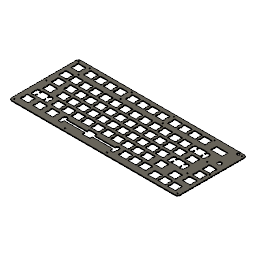
Plate (Autodesk Fusion 360 design; units mm, degrees)
part number: 2026-06-20-08-16-56-119
Autodesk Fusion 360 part; units mm, degrees
(part 1 of 6)
derive "DerivedContext1"
sketch "Sketch3" plane through (0, 0, 0) normal (0, 0, 1) x (1, 0, 0)
  line L0 (324.2389, -5.001) -> (324.612, -5.015)
  line L1 (324.612, -5.015) -> (324.9851, -5.059)
  line L2 (324.9851, -5.059) -> (325.3502, -5.132)
  line L3 (325.3502, -5.132) -> (325.71, -5.234)
  line L4 (325.71, -5.234) -> (326.0619, -5.363)
  line L5 (326.0619, -5.363) -> (326.4006, -5.52)
  line L6 (326.4006, -5.52) -> (326.726, -5.702)
  line L7 (326.726, -5.702) -> (327.0382, -5.91)
  line L8 (327.0382, -5.91) -> (327.3319, -6.142)
  line L9 (327.3319, -6.142) -> (327.6071, -6.395)
  line L10 (327.6071, -6.395) -> (327.8611, -6.67)
  line L11 (327.8611, -6.67) -> (328.0913, -6.964)
  line L12 (328.0913, -6.964) -> (328.3003, -7.275)
  line L13 (328.3003, -7.275) -> (328.4829, -7.601)
  line L14 (328.4829, -7.601) -> (328.639, -7.94)
  line L15 (328.639, -7.94) -> (328.7686, -8.291)
  line L16 (328.7686, -8.291) -> (328.8691, -8.651)
  line L17 (328.8691, -8.651) -> (328.9432, -9.018)
  line L18 (328.9432, -9.018) -> (328.9882, -9.389)
  line L19 (328.9882, -9.389) -> (329.0014, -9.763)
  line L20 (329.0014, -9.763) -> (329.0014, -133.7389)
  line L21 (329.0014, -133.7389) -> (328.9882, -134.1131)
  line L22 (328.9882, -134.1131) -> (328.9432, -134.484)
  line L23 (328.9432, -134.484) -> (328.8691, -134.851)
  line L24 (328.8691, -134.851) -> (328.7686, -135.2111)
  line L25 (328.7686, -135.2111) -> (328.639, -135.5619)
  line L26 (328.639, -135.5619) -> (328.4829, -135.9011)
  line L27 (328.4829, -135.9011) -> (328.3003, -136.2271)
  line L28 (328.3003, -136.2271) -> (328.0913, -136.538)
  line L29 (328.0913, -136.538) -> (327.8611, -136.8319)
  line L30 (327.8611, -136.8319) -> (327.6071, -137.1071)
  line L31 (327.6071, -137.1071) -> (327.3319, -137.36)
  line L32 (327.3319, -137.36) -> (327.0382, -137.5921)
  line L33 (327.0382, -137.5921) -> (326.726, -137.8)
  line L34 (326.726, -137.8) -> (326.4006, -137.9821)
  line L35 (326.4006, -137.9821) -> (326.0619, -138.139)
  line L36 (326.0619, -138.139) -> (325.71, -138.2681)
  line L37 (325.71, -138.2681) -> (325.3502, -138.3699)
  line L38 (325.3502, -138.3699) -> (324.9851, -138.443)
  line L39 (324.9851, -138.443) -> (324.612, -138.4869)
  line L40 (324.612, -138.4869) -> (324.2389, -138.502)
  line L41 (324.2389, -138.502) -> (9.763, -138.5009)
  line L42 (9.763, -138.5009) -> (9.389, -138.4869)
  line L43 (9.389, -138.4869) -> (9.018, -138.443)
  line L44 (9.018, -138.443) -> (8.651, -138.3699)
  line L45 (8.651, -138.3699) -> (8.291, -138.2681)
  line L46 (8.291, -138.2681) -> (7.94, -138.139)
  line L47 (7.94, -138.139) -> (7.601, -137.9821)
  line L48 (7.601, -137.9821) -> (7.275, -137.8)
  line L49 (7.275, -137.8) -> (6.964, -137.5921)
  line L50 (6.964, -137.5921) -> (6.67, -137.36)
  line L51 (6.67, -137.36) -> (6.395, -137.1071)
  line L52 (6.395, -137.1071) -> (6.142, -136.8319)
  line L53 (6.142, -136.8319) -> (5.91, -136.538)
  line L54 (5.91, -136.538) -> (5.702, -136.2271)
  line L55 (5.702, -136.2271) -> (5.52, -135.9011)
  line L56 (5.52, -135.9011) -> (5.363, -135.5619)
  line L57 (5.363, -135.5619) -> (5.234, -135.2111)
  line L58 (5.234, -135.2111) -> (5.132, -134.851)
  line L59 (5.132, -134.851) -> (5.059, -134.484)
  line L60 (5.059, -134.484) -> (5.015, -134.1131)
  line L61 (5.015, -134.1131) -> (5, -133.7389)
  line L62 (5, -133.7389) -> (5.001, -9.763)
  line L63 (5.001, -9.763) -> (5.015, -9.389)
  line L64 (5.015, -9.389) -> (5.059, -9.018)
  line L65 (5.059, -9.018) -> (5.132, -8.651)
  line L66 (5.132, -8.651) -> (5.234, -8.291)
  line L67 (5.234, -8.291) -> (5.363, -7.94)
  line L68 (5.363, -7.94) -> (5.52, -7.601)
  line L69 (5.52, -7.601) -> (5.702, -7.275)
  line L70 (5.702, -7.275) -> (5.91, -6.964)
  line L71 (5.91, -6.964) -> (6.142, -6.67)
  line L72 (6.142, -6.67) -> (6.395, -6.395)
  line L73 (6.395, -6.395) -> (6.67, -6.142)
  line L74 (6.67, -6.142) -> (6.964, -5.91)
  line L75 (6.964, -5.91) -> (7.275, -5.702)
  line L76 (7.275, -5.702) -> (7.601, -5.52)
  line L77 (7.601, -5.52) -> (7.94, -5.363)
  line L78 (7.94, -5.363) -> (8.291, -5.234)
  line L79 (8.291, -5.234) -> (8.651, -5.132)
  line L80 (8.651, -5.132) -> (9.018, -5.059)
  line L81 (9.018, -5.059) -> (9.389, -5.015)
  line L82 (9.389, -5.015) -> (9.763, -5)
  line L83 (9.763, -5) -> (324.2389, -5.001)
  line L84 (264.8506, -117.2131) -> (264.8506, -118.2129)
  line L85 (264.8506, -118.2129) -> (264.0499, -118.2129)
  line L86 (264.0499, -118.2129) -> (264.0499, -121.163)
  line L87 (264.0499, -121.163) -> (264.8506, -121.163)
  line L88 (264.8506, -121.163) -> (264.8506, -127.113)
  line L89 (264.8506, -127.113) -> (264.0499, -127.113)
  line L90 (264.0499, -127.113) -> (264.0499, -130.0631)
  line L91 (264.0499, -130.0631) -> (264.8506, -130.0631)
  line L92 (264.8506, -130.0631) -> (264.8506, -131.0629)
  line L93 (264.8506, -131.0629) -> (278.7015, -131.0629)
  line L94 (278.7015, -131.0629) -> (278.7015, -130.0631)
  line L95 (278.7015, -130.0631) -> (279.5005, -130.0631)
  line L96 (279.5005, -130.0631) -> (279.5005, -127.113)
  line L97 (279.5005, -127.113) -> (278.7015, -127.113)
  line L98 (278.7015, -127.113) -> (278.7015, -121.163)
  line L99 (278.7015, -121.163) -> (279.5005, -121.163)
  line L100 (279.5005, -121.163) -> (279.5005, -118.2129)
  line L101 (279.5005, -118.2129) -> (278.7015, -118.2129)
  line L102 (278.7015, -118.2129) -> (278.7015, -117.2131)
  line L103 (278.7015, -117.2131) -> (264.8506, -117.2131)
  line L104 (283.9006, -117.2131) -> (283.9006, -118.2129)
  line L105 (283.9006, -118.2129) -> (283.0989, -118.2129)
  line L106 (283.0989, -118.2129) -> (283.0989, -121.163)
  line L107 (283.0989, -121.163) -> (283.9006, -121.163)
  line L108 (283.9006, -121.163) -> (283.9006, -127.113)
  line L109 (283.9006, -127.113) -> (283.0989, -127.113)
  line L110 (283.0989, -127.113) -> (283.0989, -130.0631)
  line L111 (283.0989, -130.0631) -> (283.9006, -130.0631)
  line L112 (283.9006, -130.0631) -> (283.9006, -131.0629)
  line L113 (283.9006, -131.0629) -> (297.7515, -131.0629)
  line L114 (297.7515, -131.0629) -> (297.7515, -130.0631)
  line L115 (297.7515, -130.0631) -> (298.5505, -130.0631)
  line L116 (298.5505, -130.0631) -> (298.5505, -127.113)
  line L117 (298.5505, -127.113) -> (297.7515, -127.113)
  line L118 (297.7515, -127.113) -> (297.7515, -121.163)
  line L119 (297.7515, -121.163) -> (298.5505, -121.163)
  line L120 (298.5505, -121.163) -> (298.5505, -118.2129)
  line L121 (298.5505, -118.2129) -> (297.7515, -118.2129)
  line L122 (297.7515, -118.2129) -> (297.7515, -117.2131)
  line L123 (297.7515, -117.2131) -> (283.9006, -117.2131)
  line L124 (302.9506, -117.2131) -> (302.9506, -118.2129)
  line L125 (302.9506, -118.2129) -> (302.1515, -118.2129)
  line L126 (302.1515, -118.2129) -> (302.1515, -121.163)
  line L127 (302.1515, -121.163) -> (302.9506, -121.163)
  line L128 (302.9506, -121.163) -> (302.9506, -127.113)
  line L129 (302.9506, -127.113) -> (302.1515, -127.113)
  line L130 (302.1515, -127.113) -> (302.1515, -130.0631)
  line L131 (302.1515, -130.0631) -> (302.9506, -130.0631)
  line L132 (302.9506, -130.0631) -> (302.9506, -131.0629)
  line L133 (302.9506, -131.0629) -> (316.8015, -131.0629)
  line L134 (316.8015, -131.0629) -> (316.8015, -130.0631)
  line L135 (316.8015, -130.0631) -> (317.6005, -130.0631)
  line L136 (317.6005, -130.0631) -> (317.6005, -127.113)
  line L137 (317.6005, -127.113) -> (316.8015, -127.113)
  line L138 (316.8015, -127.113) -> (316.8015, -121.163)
  line L139 (316.8015, -121.163) -> (317.6005, -121.163)
  line L140 (317.6005, -121.163) -> (317.6005, -118.2129)
  line L141 (317.6005, -118.2129) -> (316.8015, -118.2129)
  line L142 (316.8015, -118.2129) -> (316.8015, -117.2131)
  line L143 (316.8015, -117.2131) -> (302.9506, -117.2131)
  line L144 (133.8821, -112.4511) -> (133.8821, -113.4509)
  line L145 (133.8821, -113.4509) -> (133.082, -113.4509)
  line L146 (133.082, -113.4509) -> (133.082, -116.4011)
  line L147 (133.082, -116.4011) -> (133.8821, -116.4011)
  line L148 (133.8821, -116.4011) -> (133.8821, -117.1509)
  line L149 (133.8821, -117.1509) -> (94.107, -117.1509)
  line L150 (94.107, -117.1509) -> (94.107, -113.9211)
  line L151 (94.107, -113.9211) -> (92.3819, -113.9211)
  line L152 (92.3819, -113.9211) -> (92.3819, -113.0009)
  line L153 (92.3819, -113.0009) -> (89.2321, -113.0009)
  line L154 (89.2321, -113.0009) -> (89.2321, -113.9211)
  line L155 (89.2321, -113.9211) -> (87.507, -113.9211)
  line L156 (87.507, -113.9211) -> (87.507, -117.1509)
  line L157 (87.507, -117.1509) -> (86.682, -117.1509)
  line L158 (86.682, -117.1509) -> (86.682, -119.8009)
  line L159 (86.682, -119.8009) -> (87.507, -119.8009)
  line L160 (87.507, -119.8009) -> (87.507, -126.0711)
  line L161 (87.507, -126.0711) -> (89.2321, -126.0711)
  line L162 (89.2321, -126.0711) -> (89.2321, -127.0511)
  line L163 (89.2321, -127.0511) -> (92.3819, -127.0511)
  line L164 (92.3819, -127.0511) -> (92.3819, -126.0711)
  line L165 (92.3819, -126.0711) -> (94.107, -126.0711)
  line L166 (94.107, -126.0711) -> (94.107, -121.6009)
  line L167 (94.107, -121.6009) -> (133.8821, -121.6009)
  line L168 (133.8821, -121.6009) -> (133.8821, -122.351)
  line L169 (133.8821, -122.351) -> (133.082, -122.351)
  line L170 (133.082, -122.351) -> (133.082, -125.3011)
  line L171 (133.082, -125.3011) -> (133.8821, -125.3011)
  line L172 (133.8821, -125.3011) -> (133.8821, -126.301)
  line L173 (133.8821, -126.301) -> (147.732, -126.301)
  line L174 (147.732, -126.301) -> (147.732, -125.3011)
  line L175 (147.732, -125.3011) -> (148.5321, -125.3011)
  line L176 (148.5321, -125.3011) -> (148.5321, -122.351)
  line L177 (148.5321, -122.351) -> (147.732, -122.351)
  line L178 (147.732, -122.351) -> (147.732, -121.6009)
  line L179 (147.732, -121.6009) -> (187.507, -121.6009)
  line L180 (187.507, -121.6009) -> (187.507, -126.0711)
  line L181 (187.507, -126.0711) -> (189.2321, -126.0711)
  line L182 (189.2321, -126.0711) -> (189.2321, -127.0511)
  line L183 (189.2321, -127.0511) -> (192.382, -127.0511)
  line L184 (192.382, -127.0511) -> (192.382, -126.0711)
  line L185 (192.382, -126.0711) -> (194.1071, -126.0711)
  line L186 (194.1071, -126.0711) -> (194.1071, -119.8009)
  line L187 (194.1071, -119.8009) -> (194.932, -119.8009)
  line L188 (194.932, -119.8009) -> (194.932, -117.1509)
  line L189 (194.932, -117.1509) -> (194.1071, -117.1509)
  line L190 (194.1071, -117.1509) -> (194.1071, -113.9211)
  line L191 (194.1071, -113.9211) -> (192.382, -113.9211)
  line L192 (192.382, -113.9211) -> (192.382, -113.0009)
  line L193 (192.382, -113.0009) -> (189.2321, -113.0009)
  line L194 (189.2321, -113.0009) -> (189.2321, -113.9211)
  line L195 (189.2321, -113.9211) -> (187.507, -113.9211)
  line L196 (187.507, -113.9211) -> (187.507, -117.1509)
  line L197 (187.507, -117.1509) -> (147.732, -117.1509)
  line L198 (147.732, -117.1509) -> (147.732, -116.4011)
  line L199 (147.732, -116.4011) -> (148.5321, -116.4011)
  line L200 (148.5321, -116.4011) -> (148.5321, -113.4509)
  line L201 (148.5321, -113.4509) -> (147.732, -113.4509)
  line L202 (147.732, -113.4509) -> (147.732, -112.4511)
  line L203 (147.732, -112.4511) -> (133.8821, -112.4511)
  line L204 (14.819, -112.4511) -> (14.819, -113.4509)
  line L205 (14.819, -113.4509) -> (14.019, -113.4509)
  line L206 (14.019, -113.4509) -> (14.019, -116.4011)
  line L207 (14.019, -116.4011) -> (14.819, -116.4011)
  line L208 (14.819, -116.4011) -> (14.819, -122.351)
  line L209 (14.819, -122.351) -> (14.019, -122.351)
  line L210 (14.019, -122.351) -> (14.019, -125.3011)
  line L211 (14.019, -125.3011) -> (14.819, -125.3011)
  line L212 (14.819, -125.3011) -> (14.819, -126.301)
  line L213 (14.819, -126.301) -> (28.6689, -126.301)
  line L214 (28.6689, -126.301) -> (28.6689, -125.3011)
  line L215 (28.6689, -125.3011) -> (29.469, -125.3011)
  line L216 (29.469, -125.3011) -> (29.469, -122.351)
  line L217 (29.469, -122.351) -> (28.6689, -122.351)
  line L218 (28.6689, -122.351) -> (28.6689, -116.4011)
  line L219 (28.6689, -116.4011) -> (29.469, -116.4011)
  line L220 (29.469, -116.4011) -> (29.469, -113.4509)
  line L221 (29.469, -113.4509) -> (28.6689, -113.4509)
  line L222 (28.6689, -113.4509) -> (28.6689, -112.4511)
  line L223 (28.6689, -112.4511) -> (14.819, -112.4511)
  line L224 (38.6321, -112.4511) -> (38.6321, -113.4509)
  line L225 (38.6321, -113.4509) -> (37.832, -113.4509)
  line L226 (37.832, -113.4509) -> (37.832, -116.4011)
  line L227 (37.832, -116.4011) -> (38.6321, -116.4011)
  line L228 (38.6321, -116.4011) -> (38.6321, -122.351)
  line L229 (38.6321, -122.351) -> (37.832, -122.351)
  line L230 (37.832, -122.351) -> (37.832, -125.3011)
  line L231 (37.832, -125.3011) -> (38.6321, -125.3011)
  line L232 (38.6321, -125.3011) -> (38.6321, -126.301)
  line L233 (38.6321, -126.301) -> (52.482, -126.301)
  line L234 (52.482, -126.301) -> (52.482, -125.3011)
  line L235 (52.482, -125.3011) -> (53.2821, -125.3011)
  line L236 (53.2821, -125.3011) -> (53.2821, -122.351)
  line L237 (53.2821, -122.351) -> (52.482, -122.351)
  line L238 (52.482, -122.351) -> (52.482, -116.4011)
  line L239 (52.482, -116.4011) -> (53.2821, -116.4011)
  line L240 (53.2821, -116.4011) -> (53.2821, -113.4509)
  line L241 (53.2821, -113.4509) -> (52.482, -113.4509)
  line L242 (52.482, -113.4509) -> (52.482, -112.4511)
  line L243 (52.482, -112.4511) -> (38.6321, -112.4511)
  line L244 (62.444, -112.4511) -> (62.444, -113.4509)
  line L245 (62.444, -113.4509) -> (61.6439, -113.4509)
  line L246 (61.6439, -113.4509) -> (61.6439, -116.4011)
  line L247 (61.6439, -116.4011) -> (62.444, -116.4011)
  line L248 (62.444, -116.4011) -> (62.444, -122.351)
  line L249 (62.444, -122.351) -> (61.6439, -122.351)
  line L250 (61.6439, -122.351) -> (61.6439, -125.3011)
  line L251 (61.6439, -125.3011) -> (62.444, -125.3011)
  line L252 (62.444, -125.3011) -> (62.444, -126.301)
  line L253 (62.444, -126.301) -> (76.2939, -126.301)
  line L254 (76.2939, -126.301) -> (76.2939, -125.3011)
  line L255 (76.2939, -125.3011) -> (77.094, -125.3011)
  line L256 (77.094, -125.3011) -> (77.094, -122.351)
  line L257 (77.094, -122.351) -> (76.2939, -122.351)
  line L258 (76.2939, -122.351) -> (76.2939, -116.4011)
  line L259 (76.2939, -116.4011) -> (77.094, -116.4011)
  line L260 (77.094, -116.4011) -> (77.094, -113.4509)
  line L261 (77.094, -113.4509) -> (76.2939, -113.4509)
  line L262 (76.2939, -113.4509) -> (76.2939, -112.4511)
  line L263 (76.2939, -112.4511) -> (62.444, -112.4511)
  line L264 (202.9381, -112.4511) -> (202.9381, -113.4509)
  line L265 (202.9381, -113.4509) -> (202.138, -113.4509)
  line L266 (202.138, -113.4509) -> (202.138, -116.4011)
  line L267 (202.138, -116.4011) -> (202.9381, -116.4011)
  line L268 (202.9381, -116.4011) -> (202.9381, -122.351)
  line L269 (202.9381, -122.351) -> (202.138, -122.351)
  line L270 (202.138, -122.351) -> (202.138, -125.3011)
  line L271 (202.138, -125.3011) -> (202.9381, -125.3011)
  line L272 (202.9381, -125.3011) -> (202.9381, -126.301)
  line L273 (202.9381, -126.301) -> (216.7879, -126.301)
  line L274 (216.7879, -126.301) -> (216.7879, -125.3011)
  line L275 (216.7879, -125.3011) -> (217.588, -125.3011)
  line L276 (217.588, -125.3011) -> (217.588, -122.351)
  line L277 (217.588, -122.351) -> (216.7879, -122.351)
  line L278 (216.7879, -122.351) -> (216.7879, -116.4011)
  line L279 (216.7879, -116.4011) -> (217.588, -116.4011)
  line L280 (217.588, -116.4011) -> (217.588, -113.4509)
  line L281 (217.588, -113.4509) -> (216.7879, -113.4509)
  line L282 (216.7879, -113.4509) -> (216.7879, -112.4511)
  line L283 (216.7879, -112.4511) -> (202.9381, -112.4511)
  line L284 (221.9881, -112.4511) -> (221.9881, -113.4509)
  line L285 (221.9881, -113.4509) -> (221.188, -113.4509)
  line L286 (221.188, -113.4509) -> (221.188, -116.4011)
  line L287 (221.188, -116.4011) -> (221.9881, -116.4011)
  line L288 (221.9881, -116.4011) -> (221.9881, -122.351)
  line L289 (221.9881, -122.351) -> (221.188, -122.351)
  line L290 (221.188, -122.351) -> (221.188, -125.3011)
  line L291 (221.188, -125.3011) -> (221.9881, -125.3011)
  line L292 (221.9881, -125.3011) -> (221.9881, -126.301)
  line L293 (221.9881, -126.301) -> (235.8379, -126.301)
  line L294 (235.8379, -126.301) -> (235.8379, -125.3011)
  line L295 (235.8379, -125.3011) -> (236.638, -125.3011)
  line L296 (236.638, -125.3011) -> (236.638, -122.351)
  line L297 (236.638, -122.351) -> (235.8379, -122.351)
  line L298 (235.8379, -122.351) -> (235.8379, -116.4011)
  line L299 (235.8379, -116.4011) -> (236.638, -116.4011)
  line L300 (236.638, -116.4011) -> (236.638, -113.4509)
  line L301 (236.638, -113.4509) -> (235.8379, -113.4509)
  line L302 (235.8379, -113.4509) -> (235.8379, -112.4511)
  line L303 (235.8379, -112.4511) -> (221.9881, -112.4511)
  line L304 (241.0381, -112.4511) -> (241.0381, -113.4509)
  line L305 (241.0381, -113.4509) -> (240.238, -113.4509)
  line L306 (240.238, -113.4509) -> (240.238, -116.4011)
  line L307 (240.238, -116.4011) -> (241.0381, -116.4011)
  line L308 (241.0381, -116.4011) -> (241.0381, -122.351)
  line L309 (241.0381, -122.351) -> (240.238, -122.351)
  line L310 (240.238, -122.351) -> (240.238, -125.3011)
  line L311 (240.238, -125.3011) -> (241.0381, -125.3011)
  line L312 (241.0381, -125.3011) -> (241.0381, -126.301)
  line L313 (241.0381, -126.301) -> (254.8879, -126.301)
  line L314 (254.8879, -126.301) -> (254.8879, -125.3011)
  line L315 (254.8879, -125.3011) -> (255.688, -125.3011)
  line L316 (255.688, -125.3011) -> (255.688, -122.351)
  line L317 (255.688, -122.351) -> (254.8879, -122.351)
  line L318 (254.8879, -122.351) -> (254.8879, -116.4011)
  line L319 (254.8879, -116.4011) -> (255.688, -116.4011)
  line L320 (255.688, -116.4011) -> (255.688, -113.4509)
  line L321 (255.688, -113.4509) -> (254.8879, -113.4509)
  line L322 (254.8879, -113.4509) -> (254.8879, -112.4511)
  line L323 (254.8879, -112.4511) -> (241.0381, -112.4511)
  line L324 (283.9006, -98.1631) -> (283.9006, -99.1629)
  line L325 (283.9006, -99.1629) -> (283.0989, -99.1629)
  line L326 (283.0989, -99.1629) -> (283.0989, -102.113)
  line L327 (283.0989, -102.113) -> (283.9006, -102.113)
  line L328 (283.9006, -102.113) -> (283.9006, -108.063)
  line L329 (283.9006, -108.063) -> (283.0989, -108.063)
  line L330 (283.0989, -108.063) -> (283.0989, -111.0131)
  line L331 (283.0989, -111.0131) -> (283.9006, -111.0131)
  line L332 (283.9006, -111.0131) -> (283.9006, -112.0129)
  line L333 (283.9006, -112.0129) -> (297.7515, -112.0129)
  line L334 (297.7515, -112.0129) -> (297.7515, -111.0131)
  line L335 (297.7515, -111.0131) -> (298.5505, -111.0131)
  line L336 (298.5505, -111.0131) -> (298.5505, -108.063)
  line L337 (298.5505, -108.063) -> (297.7515, -108.063)
  line L338 (297.7515, -108.063) -> (297.7515, -102.113)
  line L339 (297.7515, -102.113) -> (298.5505, -102.113)
  line L340 (298.5505, -102.113) -> (298.5505, -99.1629)
  line L341 (298.5505, -99.1629) -> (297.7515, -99.1629)
  line L342 (297.7515, -99.1629) -> (297.7515, -98.1631)
  line L343 (297.7515, -98.1631) -> (283.9006, -98.1631)
  line L344 (24.344, -93.4) -> (24.344, -94.3999)
  line L345 (24.344, -94.3999) -> (23.544, -94.3999)
  line L346 (23.544, -94.3999) -> (23.544, -97.3511)
  line L347 (23.544, -97.3511) -> (24.344, -97.3511)
  line L348 (24.344, -97.3511) -> (24.344, -98.1009)
  line L349 (24.344, -98.1009) -> (22.669, -98.1009)
  line L350 (22.669, -98.1009) -> (22.669, -94.8701)
  line L351 (22.669, -94.8701) -> (20.944, -94.8701)
  line L352 (20.944, -94.8701) -> (20.944, -93.9501)
  line L353 (20.944, -93.9501) -> (17.794, -93.9501)
  line L354 (17.794, -93.9501) -> (17.794, -94.8701)
  line L355 (17.794, -94.8701) -> (16.069, -94.8701)
  line L356 (16.069, -94.8701) -> (16.069, -98.1009)
  line L357 (16.069, -98.1009) -> (15.244, -98.1009)
  line L358 (15.244, -98.1009) -> (15.244, -100.7499)
  line L359 (15.244, -100.7499) -> (16.069, -100.7499)
  line L360 (16.069, -100.7499) -> (16.069, -107.02)
  line L361 (16.069, -107.02) -> (17.794, -107.02)
  line L362 (17.794, -107.02) -> (17.794, -108)
  line L363 (17.794, -108) -> (20.944, -108)
  line L364 (20.944, -108) -> (20.944, -107.02)
  line L365 (20.944, -107.02) -> (22.669, -107.02)
  line L366 (22.669, -107.02) -> (22.669, -102.5501)
  line L367 (22.669, -102.5501) -> (24.344, -102.5501)
  line L368 (24.344, -102.5501) -> (24.344, -103.2999)
  line L369 (24.344, -103.2999) -> (23.544, -103.2999)
  line L370 (23.544, -103.2999) -> (23.544, -106.2501)
  line L371 (23.544, -106.2501) -> (24.344, -106.2501)
  line L372 (24.344, -106.2501) -> (24.344, -107.2499)
  line L373 (24.344, -107.2499) -> (38.1939, -107.2499)
  line L374 (38.1939, -107.2499) -> (38.1939, -106.2501)
  line L375 (38.1939, -106.2501) -> (38.994, -106.2501)
  line L376 (38.994, -106.2501) -> (38.994, -103.2999)
  line L377 (38.994, -103.2999) -> (38.1939, -103.2999)
  line L378 (38.1939, -103.2999) -> (38.1939, -102.5501)
  line L379 (38.1939, -102.5501) -> (39.869, -102.5501)
  line L380 (39.869, -102.5501) -> (39.869, -107.02)
  line L381 (39.869, -107.02) -> (41.5941, -107.02)
  line L382 (41.5941, -107.02) -> (41.5941, -108)
  line L383 (41.5941, -108) -> (44.744, -108)
  line L384 (44.744, -108) -> (44.744, -107.02)
  line L385 (44.744, -107.02) -> (46.469, -107.02)
  line L386 (46.469, -107.02) -> (46.469, -100.7499)
  line L387 (46.469, -100.7499) -> (47.294, -100.7499)
  line L388 (47.294, -100.7499) -> (47.294, -98.1009)
  line L389 (47.294, -98.1009) -> (46.469, -98.1009)
  line L390 (46.469, -98.1009) -> (46.469, -94.8701)
  line L391 (46.469, -94.8701) -> (44.744, -94.8701)
  line L392 (44.744, -94.8701) -> (44.744, -93.9501)
  line L393 (44.744, -93.9501) -> (41.5941, -93.9501)
  line L394 (41.5941, -93.9501) -> (41.5941, -94.8701)
  line L395 (41.5941, -94.8701) -> (39.869, -94.8701)
  line L396 (39.869, -94.8701) -> (39.869, -98.1009)
  line L397 (39.869, -98.1009) -> (38.1939, -98.1009)
  line L398 (38.1939, -98.1009) -> (38.1939, -97.3511)
  line L399 (38.1939, -97.3511) -> (38.994, -97.3511)
  line L400 (38.994, -97.3511) -> (38.994, -94.3999)
  line L401 (38.994, -94.3999) -> (38.1939, -94.3999)
  line L402 (38.1939, -94.3999) -> (38.1939, -93.4)
  line L403 (38.1939, -93.4) -> (24.344, -93.4)
  line L404 (55.3011, -93.4) -> (55.3011, -94.3999)
  line L405 (55.3011, -94.3999) -> (54.501, -94.3999)
  line L406 (54.501, -94.3999) -> (54.501, -97.3511)
  line L407 (54.501, -97.3511) -> (55.3011, -97.3511)
  line L408 (55.3011, -97.3511) -> (55.3011, -103.2999)
  line L409 (55.3011, -103.2999) -> (54.501, -103.2999)
  line L410 (54.501, -103.2999) -> (54.501, -106.2501)
  line L411 (54.501, -106.2501) -> (55.3011, -106.2501)
  line L412 (55.3011, -106.2501) -> (55.3011, -107.2499)
  line L413 (55.3011, -107.2499) -> (69.151, -107.2499)
  line L414 (69.151, -107.2499) -> (69.151, -106.2501)
  line L415 (69.151, -106.2501) -> (69.9511, -106.2501)
  line L416 (69.9511, -106.2501) -> (69.9511, -103.2999)
  line L417 (69.9511, -103.2999) -> (69.151, -103.2999)
  line L418 (69.151, -103.2999) -> (69.151, -97.3511)
  line L419 (69.151, -97.3511) -> (69.9511, -97.3511)
  line L420 (69.9511, -97.3511) -> (69.9511, -94.3999)
  line L421 (69.9511, -94.3999) -> (69.151, -94.3999)
  line L422 (69.151, -94.3999) -> (69.151, -93.4)
  line L423 (69.151, -93.4) -> (55.3011, -93.4)
  line L424 (74.3511, -93.4) -> (74.3511, -94.3999)
  line L425 (74.3511, -94.3999) -> (73.551, -94.3999)
  line L426 (73.551, -94.3999) -> (73.551, -97.3511)
  line L427 (73.551, -97.3511) -> (74.3511, -97.3511)
  line L428 (74.3511, -97.3511) -> (74.3511, -103.2999)
  line L429 (74.3511, -103.2999) -> (73.551, -103.2999)
  line L430 (73.551, -103.2999) -> (73.551, -106.2501)
  line L431 (73.551, -106.2501) -> (74.3511, -106.2501)
  line L432 (74.3511, -106.2501) -> (74.3511, -107.2499)
  line L433 (74.3511, -107.2499) -> (88.201, -107.2499)
  line L434 (88.201, -107.2499) -> (88.201, -106.2501)
  line L435 (88.201, -106.2501) -> (89.0011, -106.2501)
  line L436 (89.0011, -106.2501) -> (89.0011, -103.2999)
  line L437 (89.0011, -103.2999) -> (88.201, -103.2999)
  line L438 (88.201, -103.2999) -> (88.201, -97.3511)
  line L439 (88.201, -97.3511) -> (89.0011, -97.3511)
  line L440 (89.0011, -97.3511) -> (89.0011, -94.3999)
  line L441 (89.0011, -94.3999) -> (88.201, -94.3999)
  line L442 (88.201, -94.3999) -> (88.201, -93.4)
  line L443 (88.201, -93.4) -> (74.3511, -93.4)
  line L444 (93.4011, -93.4) -> (93.4011, -94.3999)
  line L445 (93.4011, -94.3999) -> (92.601, -94.3999)
  line L446 (92.601, -94.3999) -> (92.601, -97.3511)
  line L447 (92.601, -97.3511) -> (93.4011, -97.3511)
  line L448 (93.4011, -97.3511) -> (93.4011, -103.2999)
  line L449 (93.4011, -103.2999) -> (92.601, -103.2999)
  line L450 (92.601, -103.2999) -> (92.601, -106.2501)
  line L451 (92.601, -106.2501) -> (93.4011, -106.2501)
  line L452 (93.4011, -106.2501) -> (93.4011, -107.2499)
  line L453 (93.4011, -107.2499) -> (107.251, -107.2499)
  line L454 (107.251, -107.2499) -> (107.251, -106.2501)
  line L455 (107.251, -106.2501) -> (108.0511, -106.2501)
  line L456 (108.0511, -106.2501) -> (108.0511, -103.2999)
  line L457 (108.0511, -103.2999) -> (107.251, -103.2999)
  line L458 (107.251, -103.2999) -> (107.251, -97.3511)
  line L459 (107.251, -97.3511) -> (108.0511, -97.3511)
  line L460 (108.0511, -97.3511) -> (108.0511, -94.3999)
  line L461 (108.0511, -94.3999) -> (107.251, -94.3999)
  line L462 (107.251, -94.3999) -> (107.251, -93.4)
  line L463 (107.251, -93.4) -> (93.4011, -93.4)
  line L464 (112.4511, -93.4) -> (112.4511, -94.3999)
  line L465 (112.4511, -94.3999) -> (111.651, -94.3999)
  line L466 (111.651, -94.3999) -> (111.651, -97.3511)
  line L467 (111.651, -97.3511) -> (112.4511, -97.3511)
  line L468 (112.4511, -97.3511) -> (112.4511, -103.2999)
  line L469 (112.4511, -103.2999) -> (111.651, -103.2999)
  line L470 (111.651, -103.2999) -> (111.651, -106.2501)
  line L471 (111.651, -106.2501) -> (112.4511, -106.2501)
  line L472 (112.4511, -106.2501) -> (112.4511, -107.2499)
  line L473 (112.4511, -107.2499) -> (126.301, -107.2499)
  line L474 (126.301, -107.2499) -> (126.301, -106.2501)
  line L475 (126.301, -106.2501) -> (127.1011, -106.2501)
  line L476 (127.1011, -106.2501) -> (127.1011, -103.2999)
  line L477 (127.1011, -103.2999) -> (126.301, -103.2999)
  line L478 (126.301, -103.2999) -> (126.301, -97.3511)
  line L479 (126.301, -97.3511) -> (127.1011, -97.3511)
  line L480 (127.1011, -97.3511) -> (127.1011, -94.3999)
  line L481 (127.1011, -94.3999) -> (126.301, -94.3999)
  line L482 (126.301, -94.3999) -> (126.301, -93.4)
  line L483 (126.301, -93.4) -> (112.4511, -93.4)
  line L484 (131.5011, -93.4) -> (131.5011, -94.3999)
  line L485 (131.5011, -94.3999) -> (130.6999, -94.3999)
  line L486 (130.6999, -94.3999) -> (130.6999, -97.3511)
  line L487 (130.6999, -97.3511) -> (131.5011, -97.3511)
  line L488 (131.5011, -97.3511) -> (131.5011, -103.2999)
  line L489 (131.5011, -103.2999) -> (130.6999, -103.2999)
  line L490 (130.6999, -103.2999) -> (130.6999, -106.2501)
  line L491 (130.6999, -106.2501) -> (131.5011, -106.2501)
  line L492 (131.5011, -106.2501) -> (131.5011, -107.2499)
  line L493 (131.5011, -107.2499) -> (145.351, -107.2499)
  line L494 (145.351, -107.2499) -> (145.351, -106.2501)
  line L495 (145.351, -106.2501) -> (146.1511, -106.2501)
  line L496 (146.1511, -106.2501) -> (146.1511, -103.2999)
  line L497 (146.1511, -103.2999) -> (145.351, -103.2999)
  line L498 (145.351, -103.2999) -> (145.351, -97.3511)
  line L499 (145.351, -97.3511) -> (146.1511, -97.3511)
  line L500 (146.1511, -97.3511) -> (146.1511, -94.3999)
  line L501 (146.1511, -94.3999) -> (145.351, -94.3999)
  line L502 (145.351, -94.3999) -> (145.351, -93.4)
  line L503 (145.351, -93.4) -> (131.5011, -93.4)
  line L504 (150.5511, -93.4) -> (150.5511, -94.3999)
  line L505 (150.5511, -94.3999) -> (149.751, -94.3999)
  line L506 (149.751, -94.3999) -> (149.751, -97.3511)
  line L507 (149.751, -97.3511) -> (150.5511, -97.3511)
  line L508 (150.5511, -97.3511) -> (150.5511, -103.2999)
  line L509 (150.5511, -103.2999) -> (149.751, -103.2999)
  line L510 (149.751, -103.2999) -> (149.751, -106.2501)
  line L511 (149.751, -106.2501) -> (150.5511, -106.2501)
  line L512 (150.5511, -106.2501) -> (150.5511, -107.2499)
  line L513 (150.5511, -107.2499) -> (164.401, -107.2499)
  line L514 (164.401, -107.2499) -> (164.401, -106.2501)
  line L515 (164.401, -106.2501) -> (165.2011, -106.2501)
  line L516 (165.2011, -106.2501) -> (165.2011, -103.2999)
  line L517 (165.2011, -103.2999) -> (164.401, -103.2999)
  line L518 (164.401, -103.2999) -> (164.401, -97.3511)
  line L519 (164.401, -97.3511) -> (165.2011, -97.3511)
  line L520 (165.2011, -97.3511) -> (165.2011, -94.3999)
  line L521 (165.2011, -94.3999) -> (164.401, -94.3999)
  line L522 (164.401, -94.3999) -> (164.401, -93.4)
  line L523 (164.401, -93.4) -> (150.5511, -93.4)
  line L524 (169.6011, -93.4) -> (169.6011, -94.3999)
  line L525 (169.6011, -94.3999) -> (168.801, -94.3999)
  line L526 (168.801, -94.3999) -> (168.801, -97.3511)
  line L527 (168.801, -97.3511) -> (169.6011, -97.3511)
  line L528 (169.6011, -97.3511) -> (169.6011, -103.2999)
  line L529 (169.6011, -103.2999) -> (168.801, -103.2999)
  line L530 (168.801, -103.2999) -> (168.801, -106.2501)
  line L531 (168.801, -106.2501) -> (169.6011, -106.2501)
  line L532 (169.6011, -106.2501) -> (169.6011, -107.2499)
  line L533 (169.6011, -107.2499) -> (183.451, -107.2499)
  line L534 (183.451, -107.2499) -> (183.451, -106.2501)
  line L535 (183.451, -106.2501) -> (184.2511, -106.2501)
  line L536 (184.2511, -106.2501) -> (184.2511, -103.2999)
  line L537 (184.2511, -103.2999) -> (183.451, -103.2999)
  line L538 (183.451, -103.2999) -> (183.451, -97.3511)
  line L539 (183.451, -97.3511) -> (184.2511, -97.3511)
  line L540 (184.2511, -97.3511) -> (184.2511, -94.3999)
  line L541 (184.2511, -94.3999) -> (183.451, -94.3999)
  line L542 (183.451, -94.3999) -> (183.451, -93.4)
  line L543 (183.451, -93.4) -> (169.6011, -93.4)
  line L544 (188.6511, -93.4) -> (188.6511, -94.3999)
  line L545 (188.6511, -94.3999) -> (187.851, -94.3999)
  line L546 (187.851, -94.3999) -> (187.851, -97.3511)
  line L547 (187.851, -97.3511) -> (188.6511, -97.3511)
  line L548 (188.6511, -97.3511) -> (188.6511, -103.2999)
  line L549 (188.6511, -103.2999) -> (187.851, -103.2999)
  line L550 (187.851, -103.2999) -> (187.851, -106.2501)
  line L551 (187.851, -106.2501) -> (188.6511, -106.2501)
  line L552 (188.6511, -106.2501) -> (188.6511, -107.2499)
  line L553 (188.6511, -107.2499) -> (202.501, -107.2499)
  line L554 (202.501, -107.2499) -> (202.501, -106.2501)
  line L555 (202.501, -106.2501) -> (203.3011, -106.2501)
  line L556 (203.3011, -106.2501) -> (203.3011, -103.2999)
  line L557 (203.3011, -103.2999) -> (202.501, -103.2999)
  line L558 (202.501, -103.2999) -> (202.501, -97.3511)
  line L559 (202.501, -97.3511) -> (203.3011, -97.3511)
  line L560 (203.3011, -97.3511) -> (203.3011, -94.3999)
  line L561 (203.3011, -94.3999) -> (202.501, -94.3999)
  line L562 (202.501, -94.3999) -> (202.501, -93.4)
  line L563 (202.501, -93.4) -> (188.6511, -93.4)
  line L564 (207.7011, -93.4) -> (207.7011, -94.3999)
  line L565 (207.7011, -94.3999) -> (206.901, -94.3999)
  line L566 (206.901, -94.3999) -> (206.901, -97.3511)
  line L567 (206.901, -97.3511) -> (207.7011, -97.3511)
  line L568 (207.7011, -97.3511) -> (207.7011, -103.2999)
  line L569 (207.7011, -103.2999) -> (206.901, -103.2999)
  line L570 (206.901, -103.2999) -> (206.901, -106.2501)
  line L571 (206.901, -106.2501) -> (207.7011, -106.2501)
  line L572 (207.7011, -106.2501) -> (207.7011, -107.2499)
  line L573 (207.7011, -107.2499) -> (221.551, -107.2499)
  line L574 (221.551, -107.2499) -> (221.551, -106.2501)
  line L575 (221.551, -106.2501) -> (222.3511, -106.2501)
  line L576 (222.3511, -106.2501) -> (222.3511, -103.2999)
  line L577 (222.3511, -103.2999) -> (221.551, -103.2999)
  line L578 (221.551, -103.2999) -> (221.551, -97.3511)
  line L579 (221.551, -97.3511) -> (222.3511, -97.3511)
  line L580 (222.3511, -97.3511) -> (222.3511, -94.3999)
  line L581 (222.3511, -94.3999) -> (221.551, -94.3999)
  line L582 (221.551, -94.3999) -> (221.551, -93.4)
  line L583 (221.551, -93.4) -> (207.7011, -93.4)
  line L584 (226.7511, -93.4) -> (226.7511, -94.3999)
  line L585 (226.7511, -94.3999) -> (225.951, -94.3999)
  line L586 (225.951, -94.3999) -> (225.951, -97.3511)
  line L587 (225.951, -97.3511) -> (226.7511, -97.3511)
  line L588 (226.7511, -97.3511) -> (226.7511, -103.2999)
  line L589 (226.7511, -103.2999) -> (225.951, -103.2999)
  line L590 (225.951, -103.2999) -> (225.951, -106.2501)
  line L591 (225.951, -106.2501) -> (226.7511, -106.2501)
  line L592 (226.7511, -106.2501) -> (226.7511, -107.2499)
  line L593 (226.7511, -107.2499) -> (240.601, -107.2499)
  line L594 (240.601, -107.2499) -> (240.601, -106.2501)
  line L595 (240.601, -106.2501) -> (241.4011, -106.2501)
  line L596 (241.4011, -106.2501) -> (241.4011, -103.2999)
  line L597 (241.4011, -103.2999) -> (240.601, -103.2999)
  line L598 (240.601, -103.2999) -> (240.601, -97.3511)
  line L599 (240.601, -97.3511) -> (241.4011, -97.3511)
  line L600 (241.4011, -97.3511) -> (241.4011, -94.3999)
  line L601 (241.4011, -94.3999) -> (240.601, -94.3999)
  line L602 (240.601, -94.3999) -> (240.601, -93.4)
  line L603 (240.601, -93.4) -> (226.7511, -93.4)
  line L604 (252.944, -93.4) -> (252.944, -94.3999)
  line L605 (252.944, -94.3999) -> (252.1439, -94.3999)
  line L606 (252.1439, -94.3999) -> (252.1439, -97.3511)
  line L607 (252.1439, -97.3511) -> (252.944, -97.3511)
  line L608 (252.944, -97.3511) -> (252.944, -103.2999)
  line L609 (252.944, -103.2999) -> (252.1439, -103.2999)
  line L610 (252.1439, -103.2999) -> (252.1439, -106.2501)
  line L611 (252.1439, -106.2501) -> (252.944, -106.2501)
  line L612 (252.944, -106.2501) -> (252.944, -107.2499)
  line L613 (252.944, -107.2499) -> (266.7952, -107.2499)
  line L614 (266.7952, -107.2499) -> (266.7952, -106.2501)
  line L615 (266.7952, -106.2501) -> (267.5943, -106.2501)
  line L616 (267.5943, -106.2501) -> (267.5943, -103.2999)
  line L617 (267.5943, -103.2999) -> (266.7952, -103.2999)
  line L618 (266.7952, -103.2999) -> (266.7952, -97.3511)
  line L619 (266.7952, -97.3511) -> (267.5943, -97.3511)
  line L620 (267.5943, -97.3511) -> (267.5943, -94.3999)
  line L621 (267.5943, -94.3999) -> (266.7952, -94.3999)
  line L622 (266.7952, -94.3999) -> (266.7952, -93.4)
  line L623 (266.7952, -93.4) -> (252.944, -93.4)
  line L624 (307.7131, -93.4) -> (307.7131, -94.3999)
  line L625 (307.7131, -94.3999) -> (306.914, -94.3999)
  line L626 (306.914, -94.3999) -> (306.914, -97.3511)
  line L627 (306.914, -97.3511) -> (307.7131, -97.3511)
  line L628 (307.7131, -97.3511) -> (307.7131, -103.2999)
  line L629 (307.7131, -103.2999) -> (306.914, -103.2999)
  line L630 (306.914, -103.2999) -> (306.914, -106.2501)
  line L631 (306.914, -106.2501) -> (307.7131, -106.2501)
  line L632 (307.7131, -106.2501) -> (307.7131, -107.2499)
  line L633 (307.7131, -107.2499) -> (321.564, -107.2499)
  line L634 (321.564, -107.2499) -> (321.564, -106.2501)
  line L635 (321.564, -106.2501) -> (322.363, -106.2501)
  line L636 (322.363, -106.2501) -> (322.363, -103.2999)
  line L637 (322.363, -103.2999) -> (321.564, -103.2999)
  line L638 (321.564, -103.2999) -> (321.564, -97.3511)
  line L639 (321.564, -97.3511) -> (322.363, -97.3511)
  line L640 (322.363, -97.3511) -> (322.363, -94.3999)
  line L641 (322.363, -94.3999) -> (321.564, -94.3999)
  line L642 (321.564, -94.3999) -> (321.564, -93.4)
  line L643 (321.564, -93.4) -> (307.7131, -93.4)
  line L644 (267.2318, -74.3511) -> (267.2318, -75.3509)
  line L645 (267.2318, -75.3509) -> (266.4328, -75.3509)
  line L646 (266.4328, -75.3509) -> (266.4328, -78.3011)
  line L647 (266.4328, -78.3011) -> (267.2318, -78.3011)
  line L648 (267.2318, -78.3011) -> (267.2318, -79.0509)
  line L649 (267.2318, -79.0509) -> (265.557, -79.0509)
  line L650 (265.557, -79.0509) -> (265.557, -75.8211)
  line L651 (265.557, -75.8211) -> (263.8319, -75.8211)
  line L652 (263.8319, -75.8211) -> (263.8319, -74.9001)
  line L653 (263.8319, -74.9001) -> (260.681, -74.9001)
  line L654 (260.681, -74.9001) -> (260.681, -75.8211)
  line L655 (260.681, -75.8211) -> (258.957, -75.8211)
  line L656 (258.957, -75.8211) -> (258.957, -79.0509)
  line L657 (258.957, -79.0509) -> (258.1309, -79.0509)
  line L658 (258.1309, -79.0509) -> (258.1309, -81.6999)
  line L659 (258.1309, -81.6999) -> (258.957, -81.6999)
  line L660 (258.957, -81.6999) -> (258.957, -87.97)
  line L661 (258.957, -87.97) -> (260.681, -87.97)
  line L662 (260.681, -87.97) -> (260.681, -88.95)
  line L663 (260.681, -88.95) -> (263.8319, -88.95)
  line L664 (263.8319, -88.95) -> (263.8319, -87.97)
  line L665 (263.8319, -87.97) -> (265.557, -87.97)
  line L666 (265.557, -87.97) -> (265.557, -83.5001)
  line L667 (265.557, -83.5001) -> (267.2318, -83.5001)
  line L668 (267.2318, -83.5001) -> (267.2318, -84.2499)
  line L669 (267.2318, -84.2499) -> (266.4328, -84.2499)
  line L670 (266.4328, -84.2499) -> (266.4328, -87.2001)
  line L671 (266.4328, -87.2001) -> (267.2318, -87.2001)
  line L672 (267.2318, -87.2001) -> (267.2318, -88.1999)
  line L673 (267.2318, -88.1999) -> (281.0827, -88.1999)
  line L674 (281.0827, -88.1999) -> (281.0827, -87.2001)
  line L675 (281.0827, -87.2001) -> (281.8818, -87.2001)
  line L676 (281.8818, -87.2001) -> (281.8818, -84.2499)
  line L677 (281.8818, -84.2499) -> (281.0827, -84.2499)
  line L678 (281.0827, -84.2499) -> (281.0827, -83.5001)
  line L679 (281.0827, -83.5001) -> (282.7575, -83.5001)
  line L680 (282.7575, -83.5001) -> (282.7575, -87.97)
  line L681 (282.7575, -87.97) -> (284.4826, -87.97)
  line L682 (284.4826, -87.97) -> (284.4826, -88.95)
  line L683 (284.4826, -88.95) -> (287.6312, -88.95)
  line L684 (287.6312, -88.95) -> (287.6312, -87.97)
  line L685 (287.6312, -87.97) -> (289.3563, -87.97)
  line L686 (289.3563, -87.97) -> (289.3563, -81.6999)
  line L687 (289.3563, -81.6999) -> (290.1818, -81.6999)
  line L688 (290.1818, -81.6999) -> (290.1818, -79.0509)
  line L689 (290.1818, -79.0509) -> (289.3563, -79.0509)
  line L690 (289.3563, -79.0509) -> (289.3563, -75.8211)
  line L691 (289.3563, -75.8211) -> (287.6312, -75.8211)
  line L692 (287.6312, -75.8211) -> (287.6312, -74.9001)
  line L693 (287.6312, -74.9001) -> (284.4826, -74.9001)
  line L694 (284.4826, -74.9001) -> (284.4826, -75.8211)
  line L695 (284.4826, -75.8211) -> (282.7575, -75.8211)
  line L696 (282.7575, -75.8211) -> (282.7575, -79.0509)
  line L697 (282.7575, -79.0509) -> (281.0827, -79.0509)
  line L698 (281.0827, -79.0509) -> (281.0827, -78.3011)
  line L699 (281.0827, -78.3011) -> (281.8818, -78.3011)
  line L700 (281.8818, -78.3011) -> (281.8818, -75.3509)
  line L701 (281.8818, -75.3509) -> (281.0827, -75.3509)
  line L702 (281.0827, -75.3509) -> (281.0827, -74.3511)
  line L703 (281.0827, -74.3511) -> (267.2318, -74.3511)
  line L704 (19.582, -74.3511) -> (19.582, -75.3509)
  line L705 (19.582, -75.3509) -> (18.782, -75.3509)
  line L706 (18.782, -75.3509) -> (18.782, -78.3011)
  line L707 (18.782, -78.3011) -> (19.582, -78.3011)
  line L708 (19.582, -78.3011) -> (19.582, -84.2499)
  line L709 (19.582, -84.2499) -> (18.782, -84.2499)
  line L710 (18.782, -84.2499) -> (18.782, -87.2001)
  line L711 (18.782, -87.2001) -> (19.582, -87.2001)
  line L712 (19.582, -87.2001) -> (19.582, -88.1999)
  line L713 (19.582, -88.1999) -> (33.432, -88.1999)
  line L714 (33.432, -88.1999) -> (33.432, -87.2001)
  line L715 (33.432, -87.2001) -> (34.2321, -87.2001)
  line L716 (34.2321, -87.2001) -> (34.2321, -84.2499)
  line L717 (34.2321, -84.2499) -> (33.432, -84.2499)
  line L718 (33.432, -84.2499) -> (33.432, -78.3011)
  line L719 (33.432, -78.3011) -> (34.2321, -78.3011)
  line L720 (34.2321, -78.3011) -> (34.2321, -75.3509)
  line L721 (34.2321, -75.3509) -> (33.432, -75.3509)
  line L722 (33.432, -75.3509) -> (33.432, -74.3511)
  line L723 (33.432, -74.3511) -> (19.582, -74.3511)
  line L724 (45.7761, -74.3511) -> (45.7761, -75.3509)
  line L725 (45.7761, -75.3509) -> (44.976, -75.3509)
  line L726 (44.976, -75.3509) -> (44.976, -78.3011)
  line L727 (44.976, -78.3011) -> (45.7761, -78.3011)
  line L728 (45.7761, -78.3011) -> (45.7761, -84.2499)
  line L729 (45.7761, -84.2499) -> (44.976, -84.2499)
  line L730 (44.976, -84.2499) -> (44.976, -87.2001)
  line L731 (44.976, -87.2001) -> (45.7761, -87.2001)
  line L732 (45.7761, -87.2001) -> (45.7761, -88.1999)
  line L733 (45.7761, -88.1999) -> (59.626, -88.1999)
  line L734 (59.626, -88.1999) -> (59.626, -87.2001)
  line L735 (59.626, -87.2001) -> (60.4261, -87.2001)
  line L736 (60.4261, -87.2001) -> (60.4261, -84.2499)
  line L737 (60.4261, -84.2499) -> (59.626, -84.2499)
  line L738 (59.626, -84.2499) -> (59.626, -78.3011)
  line L739 (59.626, -78.3011) -> (60.4261, -78.3011)
  line L740 (60.4261, -78.3011) -> (60.4261, -75.3509)
  line L741 (60.4261, -75.3509) -> (59.626, -75.3509)
  line L742 (59.626, -75.3509) -> (59.626, -74.3511)
  line L743 (59.626, -74.3511) -> (45.7761, -74.3511)
  line L744 (64.8261, -74.3511) -> (64.8261, -75.3509)
  line L745 (64.8261, -75.3509) -> (64.026, -75.3509)
  line L746 (64.026, -75.3509) -> (64.026, -78.3011)
  line L747 (64.026, -78.3011) -> (64.8261, -78.3011)
  line L748 (64.8261, -78.3011) -> (64.8261, -84.2499)
  line L749 (64.8261, -84.2499) -> (64.026, -84.2499)
  line L750 (64.026, -84.2499) -> (64.026, -87.2001)
  line L751 (64.026, -87.2001) -> (64.8261, -87.2001)
  line L752 (64.8261, -87.2001) -> (64.8261, -88.1999)
  line L753 (64.8261, -88.1999) -> (78.676, -88.1999)
  line L754 (78.676, -88.1999) -> (78.676, -87.2001)
  line L755 (78.676, -87.2001) -> (79.4761, -87.2001)
  line L756 (79.4761, -87.2001) -> (79.4761, -84.2499)
  line L757 (79.4761, -84.2499) -> (78.676, -84.2499)
  line L758 (78.676, -84.2499) -> (78.676, -78.3011)
  line L759 (78.676, -78.3011) -> (79.4761, -78.3011)
  line L760 (79.4761, -78.3011) -> (79.4761, -75.3509)
  line L761 (79.4761, -75.3509) -> (78.676, -75.3509)
  line L762 (78.676, -75.3509) -> (78.676, -74.3511)
  line L763 (78.676, -74.3511) -> (64.8261, -74.3511)
  line L764 (83.8761, -74.3511) -> (83.8761, -75.3509)
  line L765 (83.8761, -75.3509) -> (83.076, -75.3509)
  line L766 (83.076, -75.3509) -> (83.076, -78.3011)
  line L767 (83.076, -78.3011) -> (83.8761, -78.3011)
  line L768 (83.8761, -78.3011) -> (83.8761, -84.2499)
  line L769 (83.8761, -84.2499) -> (83.076, -84.2499)
  line L770 (83.076, -84.2499) -> (83.076, -87.2001)
  line L771 (83.076, -87.2001) -> (83.8761, -87.2001)
  line L772 (83.8761, -87.2001) -> (83.8761, -88.1999)
  line L773 (83.8761, -88.1999) -> (97.726, -88.1999)
  line L774 (97.726, -88.1999) -> (97.726, -87.2001)
  line L775 (97.726, -87.2001) -> (98.525, -87.2001)
  line L776 (98.525, -87.2001) -> (98.525, -84.2499)
  line L777 (98.525, -84.2499) -> (97.726, -84.2499)
  line L778 (97.726, -84.2499) -> (97.726, -78.3011)
  line L779 (97.726, -78.3011) -> (98.525, -78.3011)
  line L780 (98.525, -78.3011) -> (98.525, -75.3509)
  line L781 (98.525, -75.3509) -> (97.726, -75.3509)
  line L782 (97.726, -75.3509) -> (97.726, -74.3511)
  line L783 (97.726, -74.3511) -> (83.8761, -74.3511)
  line L784 (102.9261, -74.3511) -> (102.9261, -75.3509)
  line L785 (102.9261, -75.3509) -> (102.126, -75.3509)
  line L786 (102.126, -75.3509) -> (102.126, -78.3011)
  line L787 (102.126, -78.3011) -> (102.9261, -78.3011)
  line L788 (102.9261, -78.3011) -> (102.9261, -84.2499)
  line L789 (102.9261, -84.2499) -> (102.126, -84.2499)
  line L790 (102.126, -84.2499) -> (102.126, -87.2001)
  line L791 (102.126, -87.2001) -> (102.9261, -87.2001)
  line L792 (102.9261, -87.2001) -> (102.9261, -88.1999)
  line L793 (102.9261, -88.1999) -> (116.7749, -88.1999)
  line L794 (116.7749, -88.1999) -> (116.7749, -87.2001)
  line L795 (116.7749, -87.2001) -> (117.575, -87.2001)
  line L796 (117.575, -87.2001) -> (117.575, -84.2499)
  line L797 (117.575, -84.2499) -> (116.7749, -84.2499)
  line L798 (116.7749, -84.2499) -> (116.7749, -78.3011)
  line L799 (116.7749, -78.3011) -> (117.575, -78.3011)
  line L800 (117.575, -78.3011) -> (117.575, -75.3509)
  line L801 (117.575, -75.3509) -> (116.7749, -75.3509)
  line L802 (116.7749, -75.3509) -> (116.7749, -74.3511)
  line L803 (116.7749, -74.3511) -> (102.9261, -74.3511)
  line L804 (121.9761, -74.3511) -> (121.9761, -75.3509)
  line L805 (121.9761, -75.3509) -> (121.176, -75.3509)
  line L806 (121.176, -75.3509) -> (121.176, -78.3011)
  line L807 (121.176, -78.3011) -> (121.9761, -78.3011)
  line L808 (121.9761, -78.3011) -> (121.9761, -84.2499)
  line L809 (121.9761, -84.2499) -> (121.176, -84.2499)
  line L810 (121.176, -84.2499) -> (121.176, -87.2001)
  line L811 (121.176, -87.2001) -> (121.9761, -87.2001)
  line L812 (121.9761, -87.2001) -> (121.9761, -88.1999)
  line L813 (121.9761, -88.1999) -> (135.826, -88.1999)
  line L814 (135.826, -88.1999) -> (135.826, -87.2001)
  line L815 (135.826, -87.2001) -> (136.6261, -87.2001)
  line L816 (136.6261, -87.2001) -> (136.6261, -84.2499)
  line L817 (136.6261, -84.2499) -> (135.826, -84.2499)
  line L818 (135.826, -84.2499) -> (135.826, -78.3011)
  line L819 (135.826, -78.3011) -> (136.6261, -78.3011)
  line L820 (136.6261, -78.3011) -> (136.6261, -75.3509)
  line L821 (136.6261, -75.3509) -> (135.826, -75.3509)
  line L822 (135.826, -75.3509) -> (135.826, -74.3511)
  line L823 (135.826, -74.3511) -> (121.9761, -74.3511)
  line L824 (141.0261, -74.3511) -> (141.0261, -75.3509)
  line L825 (141.0261, -75.3509) -> (140.226, -75.3509)
  line L826 (140.226, -75.3509) -> (140.226, -78.3011)
  line L827 (140.226, -78.3011) -> (141.0261, -78.3011)
  line L828 (141.0261, -78.3011) -> (141.0261, -84.2499)
  line L829 (141.0261, -84.2499) -> (140.226, -84.2499)
  line L830 (140.226, -84.2499) -> (140.226, -87.2001)
  line L831 (140.226, -87.2001) -> (141.0261, -87.2001)
  line L832 (141.0261, -87.2001) -> (141.0261, -88.1999)
  line L833 (141.0261, -88.1999) -> (154.876, -88.1999)
  line L834 (154.876, -88.1999) -> (154.876, -87.2001)
  line L835 (154.876, -87.2001) -> (155.6761, -87.2001)
  line L836 (155.6761, -87.2001) -> (155.6761, -84.2499)
  line L837 (155.6761, -84.2499) -> (154.876, -84.2499)
  line L838 (154.876, -84.2499) -> (154.876, -78.3011)
  line L839 (154.876, -78.3011) -> (155.6761, -78.3011)
  line L840 (155.6761, -78.3011) -> (155.6761, -75.3509)
  line L841 (155.6761, -75.3509) -> (154.876, -75.3509)
  line L842 (154.876, -75.3509) -> (154.876, -74.3511)
  line L843 (154.876, -74.3511) -> (141.0261, -74.3511)
  line L844 (160.0761, -74.3511) -> (160.0761, -75.3509)
  line L845 (160.0761, -75.3509) -> (159.276, -75.3509)
  line L846 (159.276, -75.3509) -> (159.276, -78.3011)
  line L847 (159.276, -78.3011) -> (160.0761, -78.3011)
  line L848 (160.0761, -78.3011) -> (160.0761, -84.2499)
  line L849 (160.0761, -84.2499) -> (159.276, -84.2499)
  line L850 (159.276, -84.2499) -> (159.276, -87.2001)
  line L851 (159.276, -87.2001) -> (160.0761, -87.2001)
  line L852 (160.0761, -87.2001) -> (160.0761, -88.1999)
  line L853 (160.0761, -88.1999) -> (173.926, -88.1999)
  line L854 (173.926, -88.1999) -> (173.926, -87.2001)
  line L855 (173.926, -87.2001) -> (174.7261, -87.2001)
  line L856 (174.7261, -87.2001) -> (174.7261, -84.2499)
  line L857 (174.7261, -84.2499) -> (173.926, -84.2499)
  line L858 (173.926, -84.2499) -> (173.926, -78.3011)
  line L859 (173.926, -78.3011) -> (174.7261, -78.3011)
  line L860 (174.7261, -78.3011) -> (174.7261, -75.3509)
  line L861 (174.7261, -75.3509) -> (173.926, -75.3509)
  line L862 (173.926, -75.3509) -> (173.926, -74.3511)
  line L863 (173.926, -74.3511) -> (160.0761, -74.3511)
  line L864 (179.1261, -74.3511) -> (179.1261, -75.3509)
  line L865 (179.1261, -75.3509) -> (178.326, -75.3509)
  line L866 (178.326, -75.3509) -> (178.326, -78.3011)
  line L867 (178.326, -78.3011) -> (179.1261, -78.3011)
  line L868 (179.1261, -78.3011) -> (179.1261, -84.2499)
  line L869 (179.1261, -84.2499) -> (178.326, -84.2499)
  line L870 (178.326, -84.2499) -> (178.326, -87.2001)
  line L871 (178.326, -87.2001) -> (179.1261, -87.2001)
  line L872 (179.1261, -87.2001) -> (179.1261, -88.1999)
  line L873 (179.1261, -88.1999) -> (192.976, -88.1999)
  line L874 (192.976, -88.1999) -> (192.976, -87.2001)
  line L875 (192.976, -87.2001) -> (193.7761, -87.2001)
  line L876 (193.7761, -87.2001) -> (193.7761, -84.2499)
  line L877 (193.7761, -84.2499) -> (192.976, -84.2499)
  line L878 (192.976, -84.2499) -> (192.976, -78.3011)
  line L879 (192.976, -78.3011) -> (193.7761, -78.3011)
  line L880 (193.7761, -78.3011) -> (193.7761, -75.3509)
  line L881 (193.7761, -75.3509) -> (192.976, -75.3509)
  line L882 (192.976, -75.3509) -> (192.976, -74.3511)
  line L883 (192.976, -74.3511) -> (179.1261, -74.3511)
  line L884 (198.1761, -74.3511) -> (198.1761, -75.3509)
  line L885 (198.1761, -75.3509) -> (197.376, -75.3509)
  line L886 (197.376, -75.3509) -> (197.376, -78.3011)
  line L887 (197.376, -78.3011) -> (198.1761, -78.3011)
  line L888 (198.1761, -78.3011) -> (198.1761, -84.2499)
  line L889 (198.1761, -84.2499) -> (197.376, -84.2499)
  line L890 (197.376, -84.2499) -> (197.376, -87.2001)
  line L891 (197.376, -87.2001) -> (198.1761, -87.2001)
  line L892 (198.1761, -87.2001) -> (198.1761, -88.1999)
  line L893 (198.1761, -88.1999) -> (212.026, -88.1999)
  line L894 (212.026, -88.1999) -> (212.026, -87.2001)
  line L895 (212.026, -87.2001) -> (212.8261, -87.2001)
  line L896 (212.8261, -87.2001) -> (212.8261, -84.2499)